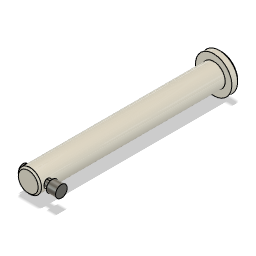
0.885.2200 - Axe pièce mobile - IGTE 21482_225065 (Autodesk Fusion 360 design; units mm, degrees)
Autodesk Fusion 360 part; units mm, degrees
sketch "Sketch1" plane through (0, 0, 0) normal (0, 0, 1) x (1, 0, 0)
  circle A0 centre (0, 0) radius 11
  dimension "d1" = 22
  constraint coincident A0.centre origin
  measures "d1" diameter of A0
extrude "Extrude1" add sketch "Sketch1" along normal blind 4.5 makes body 1
sketch "Sketch2" plane through (0, 0, 4.5) normal (0, 0, 1) x (1, 0, 0)
  circle A0 centre (0, 0) radius 11
  circle A1 centre (0, 0) radius 7
  dimension "d4" = 14
  constraint coincident A0.centre A1.centre
  measures "d4" diameter of A1
extrude "Extrude2" add sketch "Sketch2" along normal blind 112 contours A1 bodies 1
sketch "Sketch3" plane through (0, 0, 0) normal (1, 0, 0) x (0, 0, -1)
  line L0 (-116.5, 0) -> (-111.5, 0) construction
  circle A0 centre (-111.5, 0) radius 2.5
  point P0 (-116.5, 0)
  dimension "d7" = 5
  dimension "d8" = 5
  constraint coincident P0 L0.start
  constraint coincident L0.end A0.centre
  measures "d7" distance of P0 L0.end
  measures "d8" diameter of A0
extrude "Extrude3" cut sketch "Sketch3" along normal mid plane 50 bodies 1
chamfer "Chamfer1" distance 1 angle 45 1 edges at (-6.5263, -2.5313, 116.5) on bodies 1
chamfer "Chamfer2" distance 1 angle 45 1 edges at (-10.2556, -3.9778, 0) on bodies 1
sketch "Sketch4" plane through (0, 0, 0) normal (1, 0, 0) x (0, 0, -1)
  spline S0 degree 3 poles (-111.5, 2.5) (-111.1829, 2.5) (-110.8469, 2.4361) (-110.2319, 2.1801) (-109.9527, 1.9882) (-109.5119, 1.5474) (-109.3199, 1.2682) (-109.0639, 0.653) (-109, 0.3169) (-109, -0.3169) (-109.0639, -0.653) (-109.3199, -1.2682) (-109.5119, -1.5474) (-109.9527, -1.9882) (-110.2319, -2.1801) (-110.8469, -2.4361) (-111.1829, -2.5) (-111.8171, -2.5) (-112.1531, -2.4361) (-112.7681, -2.1801) (-113.0473, -1.9882) (-113.4881, -1.5474) (-113.6801, -1.2682) (-113.9361, -0.653) (-114, -0.3169) (-114, 0.3169) (-113.9361, 0.653) (-113.6801, 1.2682) (-113.4881, 1.5474) (-113.0473, 1.9882) (-112.7681, 2.1801) (-112.1531, 2.4361) (-111.8171, 2.5) (-111.5, 2.5) knots 0 0 0 0 0.095117 0.095117 0.190234 0.190234 0.285292 0.285292 0.38035 0.38035 0.475408 0.475408 0.570466 0.570466 0.665583 0.665583 0.7607 0.7607 0.855818 0.855818 0.950935 0.950935 1.045993 1.045993 1.141051 1.141051 1.236109 1.236109 1.331167 1.331167 1.426284 1.426284 1.521401 1.521401 1.521401 1.521401
  spline S1 degree 3 poles (-111.5, 2) (-111.2502, 2) (-110.9743, 1.9475) (-110.7315, 1.8465) (-110.4886, 1.7454) (-110.2596, 1.588) (-110.0858, 1.4142) (-109.9121, 1.2406) (-109.7546, 1.0114) (-109.6535, 0.7685) (-109.5525, 0.5257) (-109.5, 0.2496) (-109.5, 0) (-109.5, -0.2496) (-109.5525, -0.5257) (-109.6535, -0.7685) (-109.7546, -1.0114) (-109.9121, -1.2406) (-110.0858, -1.4142) (-110.2596, -1.588) (-110.4886, -1.7454) (-110.7315, -1.8465) (-110.9743, -1.9475) (-111.2502, -2) (-111.5, -2) (-111.7498, -2) (-112.0257, -1.9475) (-112.2685, -1.8465) (-112.5114, -1.7454) (-112.7404, -1.588) (-112.9142, -1.4142) (-113.0879, -1.2406) (-113.2454, -1.0114) (-113.3465, -0.7685) (-113.4475, -0.5257) (-113.5, -0.2496) (-113.5, 0) (-113.5, 0.2496) (-113.4475, 0.5257) (-113.3465, 0.7685) (-113.2454, 1.0114) (-113.0879, 1.2406) (-112.9142, 1.4142) (-112.7404, 1.588) (-112.5114, 1.7454) (-112.2685, 1.8465) (-112.0257, 1.9475) (-111.7498, 2) (-111.5, 2) knots 0 0 0 0 0.095117 0.095117 0.095117 0.190234 0.190234 0.190234 0.285292 0.285292 0.285292 0.38035 0.38035 0.38035 0.475408 0.475408 0.475408 0.570466 0.570466 0.570466 0.665583 0.665583 0.665583 0.7607 0.7607 0.7607 0.855818 0.855818 0.855818 0.950935 0.950935 0.950935 1.045993 1.045993 1.045993 1.141051 1.141051 1.141051 1.236109 1.236109 1.236109 1.331167 1.331167 1.331167 1.426284 1.426284 1.426284 1.521401 1.521401 1.521401 1.521401
  dimension "d13" = 0.5
  measures "d13" distance of S0
extrude "Extrude4" add sketch "Sketch4" along normal blind 15 and the other way blind 8 separate body contours S1 makes body 2
sketch "Sketch6" plane through (-8, 0, 0) normal (-1, 0, 0) x (0, 0, 1)
  spline S0 degree 3 poles (111.5, 2) (111.2502, 2) (110.9743, 1.9475) (110.7315, 1.8465) (110.4886, 1.7454) (110.2596, 1.588) (110.0858, 1.4142) (109.9121, 1.2406) (109.7546, 1.0114) (109.6535, 0.7685) (109.5525, 0.5257) (109.5, 0.2496) (109.5, 0) (109.5, -0.2496) (109.5525, -0.5257) (109.6535, -0.7685) (109.7546, -1.0114) (109.9121, -1.2406) (110.0858, -1.4142) (110.2596, -1.588) (110.4886, -1.7454) (110.7315, -1.8465) (110.9743, -1.9475) (111.2502, -2) (111.5, -2) (111.7498, -2) (112.0257, -1.9475) (112.2685, -1.8465) (112.5114, -1.7454) (112.7404, -1.588) (112.9142, -1.4142) (113.0879, -1.2406) (113.2454, -1.0114) (113.3465, -0.7685) (113.4475, -0.5257) (113.5, -0.2496) (113.5, 0) (113.5, 0.2496) (113.4475, 0.5257) (113.3465, 0.7685) (113.2454, 1.0114) (113.0879, 1.2406) (112.9142, 1.4142) (112.7404, 1.588) (112.5114, 1.7454) (112.2685, 1.8465) (112.0257, 1.9475) (111.7498, 2) (111.5, 2) knots 0 0 0 0 0.095117 0.095117 0.095117 0.190234 0.190234 0.190234 0.285292 0.285292 0.285292 0.38035 0.38035 0.38035 0.475408 0.475408 0.475408 0.570466 0.570466 0.570466 0.665583 0.665583 0.665583 0.7607 0.7607 0.7607 0.855818 0.855818 0.855818 0.950935 0.950935 0.950935 1.045993 1.045993 1.045993 1.141051 1.141051 1.141051 1.236109 1.236109 1.236109 1.331167 1.331167 1.331167 1.426284 1.426284 1.426284 1.521401 1.521401 1.521401 1.521401
  circle A0 centre (111.5, 0) radius 3
  dimension "d18" = 6
  measures "d18" diameter of A0
extrude "Extrude5" add sketch "Sketch6" against normal blind 0.95 bodies 2
sketch "Sketch7" plane through (15, 0, 0) normal (1, 0, 0) x (0, 0, -1)
  spline S0 degree 3 poles (-111.5, 2) (-111.7498, 2) (-112.0257, 1.9475) (-112.2685, 1.8465) (-112.5114, 1.7454) (-112.7404, 1.588) (-112.9142, 1.4142) (-113.0879, 1.2406) (-113.2454, 1.0114) (-113.3465, 0.7685) (-113.4475, 0.5257) (-113.5, 0.2496) (-113.5, 0) (-113.5, -0.2496) (-113.4475, -0.5257) (-113.3465, -0.7685) (-113.2454, -1.0114) (-113.0879, -1.2406) (-112.9142, -1.4142) (-112.7404, -1.588) (-112.5114, -1.7454) (-112.2685, -1.8465) (-112.0257, -1.9475) (-111.7498, -2) (-111.5, -2) (-111.2502, -2) (-110.9743, -1.9475) (-110.7315, -1.8465) (-110.4886, -1.7454) (-110.2596, -1.588) (-110.0858, -1.4142) (-109.9121, -1.2406) (-109.7546, -1.0114) (-109.6535, -0.7685) (-109.5525, -0.5257) (-109.5, -0.2496) (-109.5, 0) (-109.5, 0.2496) (-109.5525, 0.5257) (-109.6535, 0.7685) (-109.7546, 1.0114) (-109.9121, 1.2406) (-110.0858, 1.4142) (-110.2596, 1.588) (-110.4886, 1.7454) (-110.7315, 1.8465) (-110.9743, 1.9475) (-111.2502, 2) (-111.5, 2) knots -1.521401 -1.521401 -1.521401 -1.521401 -1.426284 -1.426284 -1.426284 -1.331167 -1.331167 -1.331167 -1.236109 -1.236109 -1.236109 -1.141051 -1.141051 -1.141051 -1.045993 -1.045993 -1.045993 -0.950935 -0.950935 -0.950935 -0.855818 -0.855818 -0.855818 -0.7607 -0.7607 -0.7607 -0.665583 -0.665583 -0.665583 -0.570466 -0.570466 -0.570466 -0.475408 -0.475408 -0.475408 -0.38035 -0.38035 -0.38035 -0.285292 -0.285292 -0.285292 -0.190234 -0.190234 -0.190234 -0.095117 -0.095117 -0.095117 0 0 0 0
  circle A0 centre (-111.5, 0) radius 3.5355
extrude "Extrude6" add sketch "Sketch7" against normal blind 5.5 bodies 2
named bodies: "Axe", "Goupille"
